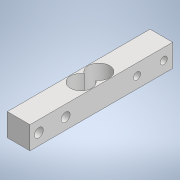
# Autodesk Inventor part: tensometr
Saved by Autodesk Inventor 2021 (Build 250183000, 183)
## iProperties
Created: 2021-11-16
Part Number: tensometr
Material: Aluminium 6061
Document SubType Name: Modeling
Designer: wojwo
Density: 2.7 g/cm^3
Appearance: Aluminium — płaski
Author: wojwo
Autodesk Inventor part; units mm, degrees
ref_plane "YZ Plane" through (0, 0, 0) normal (1, 0, 0) x (0, 1, 0)
ref_plane "XZ Plane" through (0, 0, 0) normal (0, 1, 0) x (-1, 0, 0)
ref_plane "XY Plane" through (0, 0, 0) normal (0, 0, 1) x (1, 0, 0)
sketch "Szkic1" plane through (0, 0, 0) normal (1, 0, 0) x (0, 1, 0)
  line L0 (6.35, 40) -> (-6.35, 40)
  line L1 (-6.35, 40) -> (-6.35, -40)
  line L2 (-6.35, -40) -> (6.35, -40)
  line L3 (6.35, -40) -> (6.35, 40)
  line L4 (6.35, 40) -> (-6.35, -40) construction
  line L5 (-6.35, 40) -> (6.35, -40) construction
  circle A0 centre (0, -35) radius 2
  circle A1 centre (0, -20) radius 2
  circle A2 centre (0, 20) radius 2.5
  circle A3 centre (0, 35) radius 2.5
  point P0 (0, 0)
  dimension "d0" = 12.7
  dimension "d1" = 80
  dimension "d2" = 4
  dimension "d3" = 4
  dimension "d4" = 5
  dimension "d5" = 5
  dimension "d6" = 5
  dimension "d7" = 15
  dimension "d8" = 5
  dimension "d9" = 15
  constraints: 12 end point, 4 centre point, 2 midpoint, 2 parallel, 1 horizontal, 1 perpendicular
  measures "d0" distance of L2.end L1.end
  measures "d1" distance of L1.end L0.end
  measures "d2" diameter of A0
  measures "d3" diameter of A1
  measures "d4" diameter of A2
  measures "d5" diameter of A3
  measures "d6" distance from line of L2 A0.centre
  measures "d7" distance of A0.centre A1.centre
  measures "d8" distance from line of L0 A3.centre
  measures "d9" distance of A3.centre A2.centre
extrude "Wyciągnięcie proste1" add sketch "Szkic1" along normal blind 12.7
sketch "Szkic2" plane through (0, 6.35, 40) normal (0, 1, 0) x (1, 0, 0)
  circle A0 centre (6.35, 45) radius 6
  circle A1 centre (6.35, 35) radius 6
  line L0 (12.7, 80) -> (12.7, 0) projected
  line L1 (0, 0) -> (12.7, 0) projected
  point P0 (0, 40)
  point P1 (6.35, 40)
  point P2 (9.6666, 40)
  point P3 (3.0334, 40)
  dimension "e" = 12
  dimension "d13" = 12
  dimension "d" = 10
  dimension "d15" = 6.35
  dimension "d16" = 6.35
  dimension "d17" = 5
  dimension "d18" = 40
  dimension "d19" = 6.35
  constraints: 2 centre point
  measures "e" diameter of A0
  measures "d13" diameter of A1
  measures "d" distance of A1.centre A0.centre
  measures "d15" distance from line of L0 A1.centre
  measures "d16" distance from line of L0 A0.centre
  measures "d17" distance of A1.centre point (6.35, 40)
  measures "d18" distance from line of L1 point (6.35, 40)
  measures "d19" distance from line of L0 point (6.35, 40)
extrude "Wyciągnięcie proste2" cut sketch "Szkic2" against normal through all
thread "Gwint1" size "M4x0.7" class "6H" standard "ANSI Metric M Profile" full length
thread "Gwint2" size "M4x0.7" class "6H" standard "ANSI Metric M Profile" full length
thread "Gwint3" size "M5x0.8" class "6H" standard "ANSI Metric M Profile" full length
thread "Gwint4" size "M5x0.8" class "6H" standard "ANSI Metric M Profile" full length
chamfer "Faza1" distance 0.3 angle 45 16 edges at (12.7, 6.35, 0) (6.35, 6.35, -40) (0, 6.35, 0) (6.35, 6.35, 40) (12.7, 0, 40) (0, 0, 40) (6.35, -6.35, 40) (0, -6.35, 0) (12.7, -6.35, 0) (0, 0, -40) (6.35, -6.35, -40) (12.7, 0, -40) (6.35, 6.35, -11) (6.35, 6.35, 11) (6.35, -6.35, 11) (6.35, -6.35, -11)
equation "\"d13\" = e"
equation "\"d17\" = 0.5 * d"
